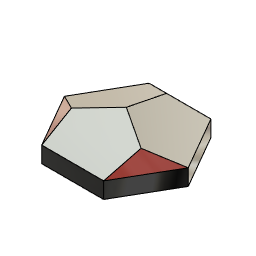
Exercise-19 v1 (Autodesk Fusion 360 design; units mm, degrees)
Autodesk Fusion 360 part; units mm, degrees
sketch "Sketch1" plane through (0, 0, 0) normal (0, 0, 1) x (1, 0, 0)
  line L0 (11.547, -0.0058) -> (5.7785, 9.9971)
  line L1 (5.7785, 9.9971) -> (-5.7685, 10.0029)
  line L2 (-5.7685, 10.0029) -> (-11.547, 0.0058)
  line L3 (-11.547, 0.0058) -> (-5.7785, -9.9971)
  line L4 (-5.7785, -9.9971) -> (5.7685, -10.0029)
  line L5 (5.7685, -10.0029) -> (11.547, -0.0058)
  dimension "d1" = 10
  measures "d1" distance of origin L5
ref_plane "WorkPlane1" through (0, 0, 4) normal (0, 0, 1) x (1, 0, 0)
sketch "Sketch2" plane through (0, 0, 4) normal (0, 0, 1) x (1, 0, 0)
  line L0 (0, 0) -> (7.5, 0) construction
  line L1 (0, 0, 0) -> (-6.4952, -3.75, -1.5)
  line L2 (0, 0, 0) -> (6.4952, -3.75, -1.5)
  line L3 (0, 0, 0) -> (0, 7.5, -1.5)
  line L4 (6.4952, -3.75, -1.5) -> (5.7685, -10.0029, -4)
  line L5 (6.4952, -3.75, -1.5) -> (11.547, -0.0058, -4)
  line L6 (0, 7.5, -1.5) -> (5.7785, 9.9971, -4)
  line L7 (-6.4952, -3.75, -1.5) -> (-5.7785, -9.9971, -4)
  line L8 (-6.4952, -3.75, -1.5) -> (-11.547, 0.0058, -4)
  line L9 (0, 7.5, -1.5) -> (-5.7685, 10.0029, -4)
  line L10 (5.7685, -10.0029, -4) -> (11.547, -0.0058, -4)
  line L11 (5.7685, -10.0029, -4) -> (-5.7785, -9.9971, -4)
  point P0 (5.7685, -10.0029)
  point P1 (11.547, -0.0058)
  point P2 (5.7785, 9.9971)
  point P3 (-5.7785, -9.9971)
  point P4 (-11.547, 0.0058)
  point P5 (-5.7685, 10.0029)
  dimension "d8" = 360
  constraint horizontal L0
  constraint coincident L0.start origin
surface "SurfacePatch1" add patch path "Sketch2" along L5 L4 L10 makes body 1
surface "SurfacePatch2" add patch path "Sketch2" along L11 L7 L1 L2 L4 separate body makes body 2
pattern_circular "C-Pattern1" count 3 over 360 about axis through (0, 0, 1.75) along (0, 0, 1) of bodies 1 2 makes body 3 at (0.0033, 9.1667, 0.8333) makes body 4 at (-7.9402, -4.5804, 0.8333) makes body 5 at (1.186, 4.2564, 2.738) makes body 6 at (-4.2792, -1.1011, 2.738)
surface "SurfacePatch3" add patch path "Sketch1" along L1 L2 L3 L4 L5 L0 separate body makes body 7
stitch "SurfaceStitch1" surfaces 1 7 4 2 6 3 5 tolerance 0.1 makes body 8
extrude "Extrude1" add 1 faces at (-1.9262, -3.3324, 0) along direction (0, 0, -1) blind 3 on bodies 8 bodies 8
